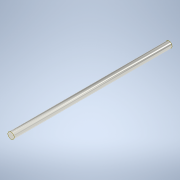
# Autodesk Inventor part: 018
Saved by Autodesk Inventor 2022.2 (Build 262287000, 287)
## iProperties
Manager: Angie Guevara
Company: ITM
Created: 2021-11-08
Part Number: 018
Material: Steel
Document SubType Name: Modeling
Designer: Samuel Gómez
Mass: 78.9168 g
Surface Area: 51.2708 cm^2
Volume: 10.0531 cm^3
Density: 7.85 g/cm^3
Appearance: Silver
Checked By: Angie Guevara
Engr Approved By: Angie Guevara
Engineer: Angie Guevara
Author: Samuel Gómez
Autodesk Inventor part; units mm, degrees
ref_plane "YZ Plane" through (0, 0, 0) normal (1, 0, 0) x (0, 1, 0)
ref_plane "XZ Plane" through (0, 0, 0) normal (0, 1, 0) x (-1, 0, 0)
ref_plane "XY Plane" through (0, 0, 0) normal (0, 0, 1) x (1, 0, 0)
sketch "Boceto1" plane through (0, 0, 0) normal (0, 0, 1) x (1, 0, 0)
  circle A0 centre (0, 0) radius 4
  dimension "d0" = 8
  constraints: 1 centre point, 1 coincident
  measures "d0" diameter of A0
extrude "Extrusión1" add sketch "Boceto1" along normal blind 200
